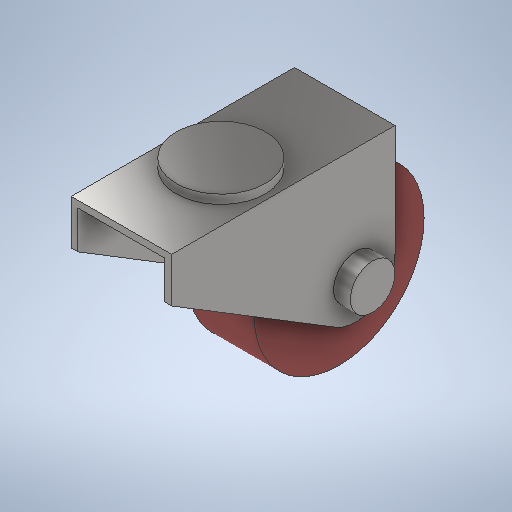
# Autodesk Inventor part: assist_wheel
Saved by Autodesk Inventor 2026.2 (Build 302298010, 298A)
## iProperties
Created: 2026-03-29
Part Number: assist_wheel
Material: Steel, Alloy
Document SubType Name: Modeling
Designer: chanh
Density: 7.73 g/cm^3
Appearance: Semi-Polished
Author: chanh
Autodesk Inventor part; units mm, degrees
ref_plane "YZ Plane" through (0, 0, 0) normal (1, 0, 0) x (0, 1, 0)
sketch "Sketch1" plane through (0, 0, 0) normal (1, 0, 0) x (0, 1, 0)
  circle A0 centre (0, 0) radius 38
  dimension "d0" = 76
  constraints: 1 centre point, 1 coincident
  measures "d0" diameter of A0
extrude "Extrusion1" add sketch "Sketch1" along normal mid plane 30
sketch "Sketch2" plane through (0, 0, 0) normal (1, 0, 0) x (0, 1, 0)
  circle A0 centre (0, 0) radius 10
  dimension "d3" = 20
  constraints: 1 centre point, 1 coincident
  measures "d3" diameter of A0
extrude "Extrusion2" add sketch "Sketch2" along normal mid plane 60
ref_plane "Work Plane1" through (22.5, 0, 0) normal (1, 0, 0) x (0, 0, -1)
sketch "Sketch3" plane through (22.5, 0, 0) normal (1, 0, 0) x (0, 0, -1)
  circle A0 centre (0, 0) radius 10 projected
  circle A1 centre (0, 0) radius 10
  circle A2 centre (0, 0) radius 17.5
  line L0 (-82.5, 50) -> (17.5, 50)
  circle A3 centre (0, 0) radius 38 projected
  line L1 (17.5, 0) -> (17.5, 50)
  line L2 (-82.5, 50) -> (-82.5, 30)
  line L3 (-82.5, 30) -> (-9.1391, -14.9241)
  point P0 (-38, 0)
  dimension "d6" = 35
  dimension "d7" = 50
  dimension "d8" = 100
  dimension "d9" = 20
  constraints: 8 end point, 2 centre point, 2 coincident, 2 horizontal alignment, 2 point on circle, 2 tangent, 2 vertical, 1 concentric, 1 horizontal, 1 other
  measures "d6" diameter of A2
  measures "d7" distance from line of point (-38, 0) L0
  measures "d8" distance between parallel lines of L1 L2
  measures "d9" distance of L0.start L2.end
extrude "Extrusion3" add sketch "Sketch3" against normal blind 3 contours A2 | A2 L3 A3 L1 | A3 L3 L2 L0 L1 picked at (-15.7584, 26.6707)
ref_plane "Work Plane2" through (-22.5, 0, 0) normal (-1, 0, 0) x (0, 0, 1)
sketch "Sketch4" plane through (-22.5, 0, 0) normal (-1, 0, 0) x (0, 0, 1)
  line L0 (9.1391, -14.9241) -> (82.5, 30) projected
  line L1 (82.5, 30) -> (82.5, 50) projected
  line L2 (82.5, 50) -> (-17.5, 50) projected
  line L3 (-17.5, 50) -> (-17.5, 0) projected
  arc A0 (-17.5, 0) -> (9.1391, -14.9241) centre (0, 0) ccw projected
  circle A1 centre (0, 0) radius 10 projected
extrude "Extrusion4" add sketch "Sketch4" against normal blind 3
sketch "Sketch5" plane through (-22.5, 50, 82.5) normal (0, 1, 0) x (1, 0, 0)
  line L0 (0, 0) -> (0, 100) projected
  line L1 (0, 0) -> (3, 0) projected
  line L2 (3, 100) -> (3, 0) projected
  line L3 (0, 100) -> (3, 100) projected
  line L4 (45, 100) -> (45, 0) projected
  line L5 (45, 100) -> (42, 100) projected
  line L6 (42, 0) -> (42, 100) projected
  line L7 (45, 0) -> (42, 0) projected
  line L8 (0, 100) -> (45, 100)
  line L9 (45, 100) -> (45, 0)
  line L10 (45, 0) -> (0, 0)
  line L11 (0, 0) -> (0, 100)
  point P0 (22.5, 82.5)
  constraints: 8 end point, 2 parallel, 1 horizontal, 1 perpendicular
extrude "Extrusion5" add sketch "Sketch5" against normal blind 3
sketch "Sketch6" plane through (22.5, 50, 82.5) normal (0, 1, 0) x (1, 0, 0)
  line L0 (-37.5, 120.5) -> (-37.5, 44.5) projected
  line L1 (-7.5, 44.5) -> (-7.5, 120.5) projected
  line L2 (-37.5, 44.5) -> (-7.5, 44.5) construction
  circle A0 centre (-22.5, 44.5) radius 20
  point P0 (-22.5, 82.5)
  dimension "d16" = 40
  constraints: 2 end point, 1 centre point, 1 midpoint, 1 perpendicular
  measures "d16" diameter of A0
extrude "Extrusion6" add sketch "Sketch6" along normal blind 4
body "Solid1"
